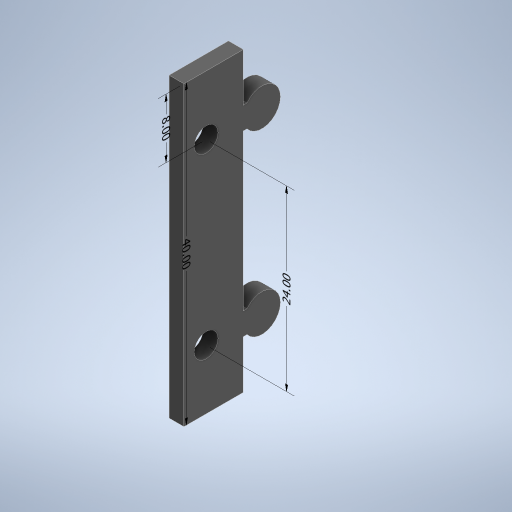
# Autodesk Inventor part: cover_setter
Saved by Autodesk Inventor 2024.1 (Build 281209000, 209)
## iProperties
Created: 2025-03-07
Part Number: cover_setter
Material: 一般
Document SubType Name: Modeling
Designer: hibik
Density: 1 g/cm^3
Appearance: 既定
Author: hibik
Autodesk Inventor part; units mm, degrees
ref_plane "YZ Plane" through (0, 0, 0) normal (1, 0, 0) x (0, 1, 0)
ref_plane "XZ Plane" through (0, 0, 0) normal (0, 1, 0) x (-1, 0, 0)
ref_plane "XY Plane" through (0, 0, 0) normal (0, 0, 1) x (1, 0, 0)
sketch "スケッチ1" plane through (0, 0, 0) normal (1, 0, 0) x (0, 1, 0)
  line L0 (20, 0) -> (0, 0)
  line L1 (0, 0) -> (0, -8)
  line L2 (0, -8) -> (20, -8)
  line L3 (20, -8) -> (20, 0)
  circle A0 centre (12, -10.5) radius 2.5 construction
  circle A1 centre (12, -10.5) radius 2.5
  line L4 (13.5, -8.5) -> (10.5, -8.5)
  line L5 (10.5, -8.5) -> (10.5, -8)
  line L6 (10.5, -8) -> (13.5, -8)
  line L7 (13.5, -8) -> (13.5, -8.5)
  line L8 (12, -10.5) -> (12, -8)
  point P0 (13.5, -8)
  point P1 (10.5, -8)
  dimension "d1" = 5
  dimension "d0" = 5
  dimension "d2" = 3
  dimension "d3" = 12
  dimension "d4" = 8
  dimension "d5" = 20
  constraints: 18 end point, 4 parallel, 3 perpendicular, 2 horizontal, 2 point on line, 1 centre point, 1 coincident, 1 collinear, 1 midpoint, 1 tangent, 4 other
  measures "d0" diameter of A0
  measures "d2" distance of L5.end L6.end
  measures "d3" horizontal distance of point (0, 0) A0.centre
  measures "d4" distance of L2.end L0.start
  measures "d5" distance of L0.start L0.end
extrude "押し出し1" add sketch "スケッチ1" along normal blind 2
mirror "ミラー1" about plane through (0, 0, 0) normal (0, -1, 0)
sketch "スケッチ2" plane through (2, 0, 0) normal (1, 0, 0) x (0, 0, -1)
  line L0 (8.5, 13.5) -> (8, 13.5) projected
  line L1 (8, 13.5) -> (8, 20) projected
  line L2 (8, 20) -> (0, 20) projected
  line L3 (0, 20) -> (0, -20) projected
  line L4 (8, -20) -> (0, -20) projected
  line L5 (8, -13.5) -> (8, -20) projected
  line L6 (8.5, -13.5) -> (8, -13.5) projected
  arc A0 (8.5, -13.5) -> (8.5, -10.5) centre (10.5, -12) ccw projected
  line L7 (8, -10.5) -> (8.5, -10.5) projected
  line L8 (8, 10.5) -> (8, -10.5) projected
  line L9 (8, 10.5) -> (8.5, 10.5) projected
  arc A1 (8.5, 10.5) -> (8.5, 13.5) centre (10.5, 12) ccw projected
  circle A2 centre (3, 12) radius 1.6
  circle A3 centre (3, -12) radius 1.6
  point P0 (0, 0)
  dimension "d8" = 3.2
  dimension "d17" = 3
  constraints: 2 centre point, 2 horizontal alignment, 1 equal radius, 1 vertical alignment
  measures "d8" diameter of A2
  measures "d17" distance from line of L3 A2.centre
extrude "押し出し2" cut sketch "スケッチ2" against normal blind 2 contours A2 | A3
